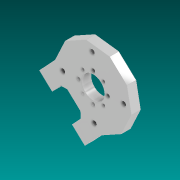
# Autodesk Inventor part: gearboxFrame
Saved by Autodesk Inventor 2020.2 (Build 242310000, 310)
## iProperties
Created: 2020-05-19
Part Number: gearboxFrame
Material: Aluminum 6061
Document SubType Name: Modeling
Designer: Svend
Density: 2.7 g/cm^3
Appearance: Aluminum - Polished
Author: Svend
Autodesk Inventor part; units mm, degrees
ref_plane "YZ Plane" through (0, 0, 0) normal (1, 0, 0) x (0, 1, 0)
ref_plane "XZ Plane" through (0, 0, 0) normal (0, 1, 0) x (-1, 0, 0)
ref_plane "XY Plane" through (0, 0, 0) normal (0, 0, 1) x (1, 0, 0)
ref_plane "Work Plane1" through (0, 0, 0) normal (0, 0, 1) x (1, 0, 0)
sketch "Sketch1" plane through (0, 0, 0) normal (0, 0, 1) x (1, 0, 0)
  circle A0 centre (0, 0) radius 12.5 projected
  circle A1 centre (0, -16) radius 2 projected
  circle A2 centre (0, 16) radius 2 projected
  circle A3 centre (-16, 0) radius 2 projected
  circle A4 centre (16, 0) radius 2 projected
  circle A5 centre (11.3137, 11.3137) radius 1.6 projected
  circle A6 centre (-11.3137, -11.3137) radius 1.6 projected
  circle A7 centre (-11.3137, 11.3137) radius 1.6 projected
  circle A8 centre (11.3137, -11.3137) radius 1.6 projected
  circle A9 centre (0, 0) radius 20.7 projected
  line L0 (31.6375, -97.9493) -> (-99.8575, 24.9697) projected
  line L1 (-23.1886, -46.699) -> (-9.2531, -59.7257) projected
  line L2 (-9.2531, -59.7257) -> (7.9751, -41.2954) projected
  line L3 (7.9751, -41.2954) -> (30.7249, -28.721) projected
  line L4 (30.7249, -28.721) -> (41.7388, -5.1762) projected
  line L5 (41.7388, -5.1762) -> (36.8098, 20.3458) projected
  line L6 (36.8098, 20.3458) -> (17.8208, 38.0964) projected
  line L7 (17.8208, 38.0964) -> (-7.9751, 41.2954) projected
  line L8 (-7.9751, 41.2954) -> (-30.7249, 28.721) projected
  line L9 (-30.7249, 28.721) -> (-41.7388, 5.1762) projected
  line L10 (-41.7388, 5.1762) -> (-58.967, -13.254) projected
  line L11 (-58.967, -13.254) -> (-45.0314, -26.2807) projected
  line L12 (-45.0314, -26.2807) -> (-35.471, -16.0534) projected
  line L13 (-28.404, -15.8151) -> (-35.471, -16.0534) projected
  line L14 (-28.404, -15.8151) -> (-13.8665, -29.4045) projected
  line L15 (-13.6283, -36.4716) -> (-13.8665, -29.4045) projected
  line L16 (-13.6283, -36.4716) -> (-23.1886, -46.699) projected
  circle A10 centre (33.3141, 1.123) radius 2.5 projected
  circle A11 centre (1.123, -33.3141) radius 2.5 projected
  circle A12 centre (0, 0) radius 21 projected
  circle A13 centre (-1.123, 33.3141) radius 2.5 projected
  circle A14 centre (-33.3141, -1.123) radius 2.5 projected
  point P0 (0, 0)
extrude "Extrusion1" add sketch "Sketch1" along normal blind 10 contours A9 | L0 L16 L15 L14 L13 L12 L10 L9 L8 L7 L6 L5 L4 L3 L2 | A12
sketch "Sketch2" plane through (-45.0314, -26.2807, 0) normal (-0.6828833, -0.7305275, 0) x (0.7305275, -0.6828833, 0)
  line L0 (-19.076, 0) -> (0, 0) projected
  line L1 (0, 0) -> (0, 10) projected
  line L2 (-19.076, 10) -> (0, 10) projected
  line L3 (-19.076, 0) -> (-19.076, 10) projected
  line L4 (29.9, 0) -> (48.976, 0) projected
  line L5 (48.976, 0) -> (48.976, 10) projected
  line L6 (29.9, 10) -> (48.976, 10) projected
  line L7 (29.9, 0) -> (29.9, 10) projected
  point P0 (14.95, 0)
  point P1 (-9.538, 5)
  point P2 (39.438, 5)
  point P3 (-19.076, 5)
  point P4 (29.9, 5)
  point P5 (39.438, 10)
  point P6 (-9.538, 10)
  constraints: 4 midpoint, 2 horizontal alignment, 2 vertical alignment
hole "Hole1" at (-51.9992, -19.7674, 5) at (-16.2209, -53.2123, 5) direction (0.6828833, 0.7305275, 0) diameter 4.917 depth 17.1 tip angle 118 thread size "M6x1" class "6H" standard "ISO Metric profile"
body "Solid1"
